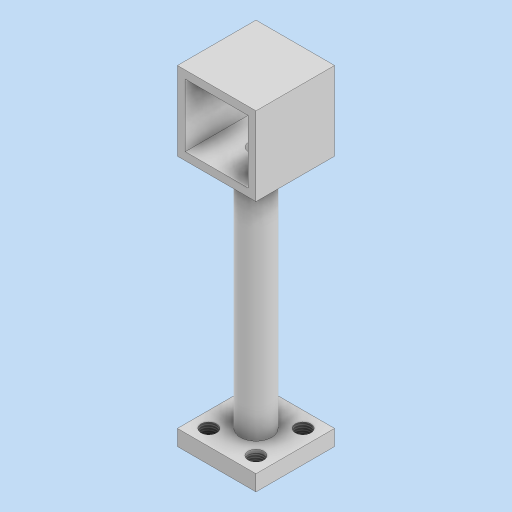
# Autodesk Inventor part: camera_pole
Saved by Autodesk Inventor 2023 (Build 270158000, 158)
## iProperties
Created: 2024-11-15
Part Number: camera_pole
Material: Generic
Document SubType Name: Modeling
Designer: ADMIN
Density: 1 g/cm^3
Appearance: Default
Author: ADMIN
Autodesk Inventor part; units mm, degrees
ref_plane "YZ Plane" through (0, 0, 0) normal (1, 0, 0) x (0, 1, 0)
ref_plane "XZ Plane" through (0, 0, 0) normal (0, 1, 0) x (-1, 0, 0)
ref_plane "XY Plane" through (0, 0, 0) normal (0, 0, 1) x (1, 0, 0)
sketch "Sketch1" plane through (0, 0, 0) normal (0, 1, 0) x (-1, 0, 0)
  line L0 (-25, 25) -> (25, 25)
  line L1 (25, 25) -> (25, -25)
  line L2 (25, -25) -> (-25, -25)
  line L3 (-25, -25) -> (-25, 25)
  line L4 (-25, 25) -> (25, -25) construction
  line L5 (25, 25) -> (-25, -25) construction
  circle A0 centre (15, -15) radius 5
  circle A1 centre (-15, -15) radius 5
  circle A2 centre (15, 15) radius 5
  circle A3 centre (-15, 15) radius 5
  circle A4 centre (0, 0) radius 10
  dimension "d0" = 50
  dimension "d1" = 50
  dimension "d2" = 10
  dimension "d3" = 10
  dimension "d6" = 30
  dimension "d9" = 30
  dimension "d12" = 20
  constraints: 12 end point, 5 centre point, 2 horizontal, 2 midpoint, 2 parallel, 1 coincident, 1 perpendicular, 1 point on line, 1 vertical, 6 other
  measures "d0" distance of L0.end L1.end
  measures "d1" distance of L1.end L2.end
  measures "d2" diameter of A0
  measures "d3" distance from line of L2 A0.centre
  measures "d6" distance of A0.centre A1.centre
  measures "d9" distance of A0.centre A2.centre
  measures "d12" diameter of A4
extrude "Extrusion1" add sketch "Sketch1" along normal blind 150 contours A4
extrude "Extrusion2" add sketch "Sketch1" against normal blind 10 contours L0 L1 L2 L3 | A4
thread "Thread1" size "M10x1.5" class "6H" standard "ANSI Metric M Profile" length 8
thread "Thread2" size "M10x1.5" class "6H" standard "ANSI Metric M Profile" length 8
thread "Thread3" size "M10x1.5" class "6H" standard "ANSI Metric M Profile" length 8
thread "Thread4" size "M10x1.5" class "6H" standard "ANSI Metric M Profile" length 8
sketch "Sketch2" plane through (0, 150, 0) normal (0, 1, 0) x (1, 0, 0)
  line L0 (25, 25) -> (-25, 25) projected
  line L1 (-25, 25) -> (-25, -25) projected
  line L2 (-25, -25) -> (25, -25) projected
  line L3 (25, -25) -> (25, 25) projected
  point P0 (0, 0)
extrude "Extrusion3" add sketch "Sketch2" along normal blind 50
shell "Shell1" thickness 5 removed faces 1 at (-8.3333, 166.6667, 25)
equation "\"d1\" = d0"
equation "\"d3\" = d2"
body "Solid1"
